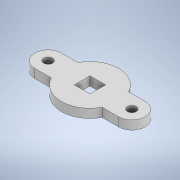
# Autodesk Inventor part: ArmBottomCap
Saved by Autodesk Inventor 2021 (Build 250183000, 183)
## iProperties
Created: 2024-01-12
Part Number: ArmBottomCap
Material: Generic
Document SubType Name: Modeling
Designer: brybr
Density: 1 g/cm^3
Appearance: Default
Author: brybr
Autodesk Inventor part; units mm, degrees
ref_plane "YZ Plane" through (0, 0, 0) normal (1, 0, 0) x (0, 1, 0)
ref_plane "XZ Plane" through (0, 0, 0) normal (0, 1, 0) x (-1, 0, 0)
ref_plane "XY Plane" through (0, 0, 0) normal (0, 0, 1) x (1, 0, 0)
sketch "Sketch1" plane through (0, 0, 0) normal (0, 1, 0) x (-1, 0, 0)
  circle A0 centre (0, 0) radius 9.7
  circle A1 centre (14.2, 0) radius 1.5
  line L0 (12.7, 0) -> (9.7, 0) construction
  line L1 (12.7, 0) -> (15.7, 0) construction
  circle A2 centre (14.2, 0) radius 4.5
  line L2 (14.2, -4.5) -> (8.593, -4.5)
  line L3 (14.2, -4.5) -> (19.807, -4.5) construction
  line L4 (14.2, 4.5) -> (8.593, 4.5)
  line L5 (14.2, 4.5) -> (19.807, 4.5) construction
  line L6 (0, 0) -> (5, 0) construction
  line L7 (0, 0) -> (0, 5) construction
  line L8 (0, 0) -> (5, 0) construction
  line L9 (-12.7, 0) -> (-9.7, 0) construction
  line L10 (-14.2, -4.5) -> (-8.593, -4.5)
  line L11 (-12.7, 0) -> (-15.7, 0) construction
  circle A3 centre (-14.2, 0) radius 1.5
  circle A4 centre (-14.2, 0) radius 4.5
  line L12 (-14.2, -4.5) -> (-19.807, -4.5) construction
  line L13 (-14.2, 4.5) -> (-19.807, 4.5) construction
  line L14 (-14.2, 4.5) -> (-8.593, 4.5)
  line L15 (2.65, -2.65) -> (2.65, 2.65)
  line L16 (2.65, 2.65) -> (-2.65, 2.65)
  line L17 (-2.65, 2.65) -> (-2.65, -2.65)
  line L18 (-2.65, -2.65) -> (2.65, -2.65)
  line L19 (2.65, -2.65) -> (-2.65, 2.65) construction
  line L20 (2.65, 2.65) -> (-2.65, -2.65) construction
  line L21 (2.65, -2.65) -> (7.95, -2.65) construction
  dimension "d1" = 3
  dimension "d0" = 19.4
  dimension "d2" = 180
  dimension "d3" = 3
  dimension "d4" = 9
  dimension "d5" = 180
  dimension "d6" = 180
  dimension "d15" = 90
  dimension "d18" = 360
  dimension "d20" = 5.3
  dimension "d21" = 90
  dimension "d22" = 5.3
  constraints: 44 end point, 7 point on circle, 6 equal length, 6 horizontal, 4 coincident, 3 centre point, 3 parallel, 3 tangent, 2 horizontal alignment, 2 midpoint, 1 perpendicular, 43 other
  measures "d0" diameter of A0
  measures "d2" angle of L0 L1
  measures "d3" distance of L0.start L0.end
  measures "d4" diameter of A2
  measures "d5" angle of L2 L3
  measures "d6" angle of L4 L5
  measures "d15" angle of L8 L7
  measures "d20" distance of L15.start L15.end
  measures "d21" angle of L21 L15
  measures "d22" distance of L16.end L15.end
extrude "Extrusion2" add sketch "Sketch1" along normal blind 3
body "Solid2"
